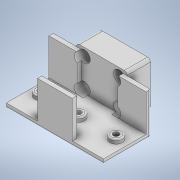
# Autodesk Inventor part: bedMount
Saved by Autodesk Inventor 2020 (Build 240168000, 168)
## iProperties
Created: 2020-01-08
Part Number: bedMount
Material: Generic
Document SubType Name: Modeling
Designer: PAB
Density: 1 g/cm^3
Appearance: Default
Author: PAB
Autodesk Inventor part; units mm, degrees
ref_plane "YZ Plane" through (0, 0, 0) normal (1, 0, 0) x (0, 1, 0)
ref_plane "XZ Plane" through (0, 0, 0) normal (0, 1, 0) x (-1, 0, 0)
ref_plane "XY Plane" through (0, 0, 0) normal (0, 0, 1) x (1, 0, 0)
sketch "Sketch1" plane through (0, 0, 0) normal (0, 1, 0) x (-1, 0, 0)
  line L0 (20.5, 16.2) -> (-20.5, 16.2)
  line L1 (-20.5, 16.2) -> (-20.5, -16.2)
  line L2 (-20.5, -16.2) -> (20.5, -16.2)
  line L3 (20.5, -16.2) -> (20.5, 16.2)
  point P0 (0, 0)
  dimension "d0" = 41
  dimension "d1" = 32.4
  constraints: 8 end point, 2 parallel, 1 horizontal, 1 perpendicular
  measures "d0" distance of L2.end L1.end
  measures "d1" distance of L1.end L0.end
extrude "Extrusion1" add sketch "Sketch1" along normal blind 3
sketch "Sketch3" plane through (0, 3, 0) normal (0, 1, 0) x (1, 0, 0)
  line L0 (-20.5, -16.2) -> (20.5, -16.2) projected
  line L1 (-20.5, 16.2) -> (-20.5, -16.2) projected
  line L2 (20.5, -16.2) -> (-20.5, -16.2)
  line L3 (-20.5, -16.2) -> (-20.5, -13.2)
  line L4 (-20.5, -13.2) -> (20.5, -13.2)
  line L5 (20.5, -13.2) -> (20.5, -16.2)
  line L6 (20.5, 16.2) -> (-20.5, 16.2) projected
  line L7 (20.5, 16.2) -> (-20.5, 16.2)
  line L8 (-20.5, 16.2) -> (-20.5, 13.2)
  line L9 (-20.5, 13.2) -> (20.5, 13.2)
  line L10 (20.5, 13.2) -> (20.5, 16.2)
  point P0 (0, 0)
  dimension "d8" = 3
  dimension "d9" = 3
  constraints: 16 end point, 4 parallel, 2 horizontal, 2 perpendicular, 2 point on line
  measures "d8" distance of L2.end L3.end
  measures "d9" distance of L8.end L7.end
extrude "Extrusion3" add sketch "Sketch3" along normal blind 25.4
sketch "Sketch4" plane through (20.5, 0, -16.2) normal (0, 0, -1) x (-1, 0, 0)
  line L0 (41, 3) -> (0, 3) projected
  line L1 (0, 28.4) -> (41, 28.4) projected
  line L2 (0, 3) -> (21.5, 3)
  line L3 (21.5, 3) -> (21.5, 28.4)
  line L4 (21.5, 28.4) -> (0, 28.4)
  line L5 (0, 28.4) -> (0, 3)
  point P0 (20.5, 0)
  dimension "d12" = 21.5
  constraints: 8 end point, 2 parallel, 1 horizontal, 1 perpendicular, 1 point on line
  measures "d12" distance of L4.end L3.end
extrude "Extrusion4" cut sketch "Sketch4" against normal blind 3
sketch "Sketch5" plane through (-20.5, 0, 16.2) normal (0, 0, 1) x (1, 0, 0)
  line L0 (41, 28.4) -> (0, 28.4) projected
  line L1 (19.5, 3) -> (41, 3) projected
  line L2 (0, 28.4) -> (21.5, 28.4)
  line L3 (21.5, 28.4) -> (21.5, 3)
  line L4 (21.5, 3) -> (0, 3)
  line L5 (0, 3) -> (0, 28.4)
  point P0 (20.5, 0)
  dimension "d15" = 21.5
  constraints: 8 end point, 2 parallel, 1 horizontal, 1 perpendicular, 1 point on line
  measures "d15" distance of L3.end L4.end
extrude "Extrusion5" cut sketch "Sketch5" against normal blind 3
sketch "Sketch6" plane through (0, 3, 0) normal (0, 1, 0) x (1, 0, 0)
  circle A0 centre (13, 0) radius 4.25
  circle A1 centre (-13, 0) radius 4.25
  line L0 (-20.5, 13.2) -> (-20.5, -16.2) projected
  line L1 (20.5, -13.2) -> (20.5, 16.2) projected
  point P0 (0, 0)
  dimension "d20" = 8.5
  dimension "d21" = 8.5
  dimension "d32" = 26
  dimension "d33" = 7.5
  dimension "d34" = 7.5
  constraints: 2 centre point
  measures "d20" diameter of A0
  measures "d21" diameter of A1
  measures "d32" distance of A0.centre A1.centre
  measures "d33" distance from line of L0 A1.centre
  measures "d34" distance from line of L1 A0.centre
extrude "Extrusion6" add sketch "Sketch6" along normal blind 3
sketch "Sketch9" plane through (20.5, 0, 16.2) normal (1, 0, 0) x (0, 0, -1)
  line L0 (32.4, 0) -> (32.4, 3) projected
  line L1 (32.4, 3) -> (0, 3)
  line L2 (0, 3) -> (0, 0)
  line L3 (0, 0) -> (32.4, 0)
  line L4 (32.4, 0) -> (32.4, 3)
  point P0 (16.2, 0)
  constraints: 8 end point, 2 parallel, 1 horizontal, 1 perpendicular
extrude "Extrusion9" add sketch "Sketch9" along normal blind 26
sketch "Sketch10" plane through (0, 3, 0) normal (0, 1, 0) x (1, 0, 0)
  circle A0 centre (39, 0) radius 4.25
  point P0 (0, 0)
  dimension "d37" = 8.5
  constraints: 1 centre point
  measures "d37" diameter of A0
extrude "Extrusion10" add sketch "Sketch10" along normal blind 3
sketch "Sketch11" plane through (0, 3, 0) normal (0, 1, 0) x (1, 0, 0)
  line L0 (46.5, 16.2) -> (46.5, -16.2) projected
  line L1 (46.5, 16.2) -> (27, 16.2)
  line L2 (27, 16.2) -> (27, 13.2)
  line L3 (27, 13.2) -> (46.5, 13.2)
  line L4 (46.5, 13.2) -> (46.5, 16.2)
  point P0 (0, 0)
  dimension "d40" = 19.5
  dimension "d41" = 3
  constraints: 8 end point, 2 parallel, 1 horizontal, 1 perpendicular
  measures "d40" distance of L3.end L2.end
  measures "d41" distance of L2.end L1.end
extrude "Extrusion11" add sketch "Sketch11" along normal blind 25.4
sketch "Sketch14" plane through (20.5, 3, 13.2) normal (1, 0, 0) x (0, 0, -1)
  line L0 (0, 0) -> (0, 25.4) projected
  line L1 (-3, 0) -> (-3, 25.4) projected
  line L2 (0, 25.4) -> (-3, 25.4)
  line L3 (-3, 25.4) -> (-3, 0)
  line L4 (-3, 0) -> (0, 0)
  line L5 (0, 0) -> (0, 25.4)
  point P0 (13.2, -3)
  constraints: 8 end point, 2 parallel, 1 horizontal, 1 perpendicular
extrude "Extrusion14" add sketch "Sketch14" along normal blind 4.5
fillet "Fillet1" radius 1 3 edges at (-17.25, 6, 0) (8.75, 6, 0) (34.75, 6, 0)
fillet "Fillet2" radius 1 6 edges at (-20.5, 14.2, -16.2) (-20.5, 0, 0) (13, 0, 16.2) (46.5, 0, 0) (46.5, 14.2, -16.2) (13, 0, -16.2)
sketch "Sketch15" plane through (0, 0, 0) normal (0, -1, 0) x (1, 0, 0)
  circle A0 centre (39, 0) radius 4.25 projected
  circle A1 centre (39, 0) radius 2
  circle A2 centre (13, 0) radius 3.25 projected
  circle A3 centre (13, 0) radius 2
  circle A4 centre (-13, 0) radius 3.25 projected
  circle A5 centre (-13, 0) radius 2
  point P0 (0, 0)
  dimension "d54" = 4
  dimension "d55" = 4
  dimension "d56" = 4
  constraints: 3 centre point, 3 coincident
  measures "d54" diameter of A1
  measures "d55" diameter of A3
  measures "d56" diameter of A5
extrude "Extrusion15" cut sketch "Sketch15" against normal blind 10 contours A1 | A3 | A5
sketch "Sketch16" plane through (0, 0, 0) normal (0, -1, 0) x (1, 0, 0)
  circle A0 centre (39, 0) radius 2 projected
  circle A1 centre (39, 0) radius 3
  circle A2 centre (13, 0) radius 2 projected
  circle A3 centre (13, 0) radius 3
  circle A4 centre (-13, 0) radius 2 projected
  circle A5 centre (-13, 0) radius 3
  point P0 (0, 0)
  dimension "d59" = 6
  dimension "d60" = 6
  dimension "d61" = 6
  constraints: 3 centre point, 3 coincident
  measures "d59" diameter of A1
  measures "d60" diameter of A3
  measures "d61" diameter of A5
extrude "Extrusion16" cut sketch "Sketch16" against normal blind 3 contours A0 | A1 | A2 | A3 | A4 | A5
sketch "Sketch17" plane through (-1, 3, -16.2) normal (0, 0, -1) x (-1, 0, 0)
  line L0 (3.5, 27.7) -> (-31.5, 27.7)
  line L1 (-31.5, 27.7) -> (-31.5, -2.3)
  line L2 (-31.5, -2.3) -> (3.5, -2.3)
  line L3 (3.5, -2.3) -> (3.5, 27.7)
  point P0 (-1, -3)
  dimension "d64" = 35
  dimension "d65" = 30
  constraints: 8 end point, 2 parallel, 1 horizontal, 1 perpendicular
  measures "d64" distance of L2.end L1.end
  measures "d65" distance of L1.end L0.end
extrude "Extrusion17" add sketch "Sketch17" along normal blind 16
sketch "Sketch18" plane through (-1, 3, -32.2) normal (0, 0, -1) x (-1, 0, 0)
  line L0 (-31.5, -2) -> (-31.5, -2.3) projected
  line L1 (0, 0) -> (19.5, 0) projected
  line L2 (-31.5, -2.3) -> (3.5, -2.3)
  line L3 (3.5, -2.3) -> (3.5, 0)
  line L4 (3.5, 0) -> (-31.5, 0)
  line L5 (-31.5, 0) -> (-31.5, -2.3)
  point P0 (-1, -3)
  dimension "d68" = 35
  constraints: 8 end point, 2 parallel, 1 horizontal, 1 perpendicular, 1 point on line
  measures "d68" distance of L4.end L3.end
extrude "Extrusion19" add sketch "Sketch18" against normal blind 19
sketch "Sketch19" plane through (-20.5, 3, -13.2) normal (0, 0, 1) x (1, 0, 0)
  circle A0 centre (45.5, 22.35) radius 4
  circle A1 centre (21.5, 22.35) radius 4
  line L0 (45.5, 25.4) -> (45.5, 0) projected
  circle A2 centre (45.5, 3.35) radius 4
  line L1 (21.5, 0) -> (21.5, 25.4) projected
  circle A3 centre (21.5, 3.35) radius 4
  point P0 (20.5, -3)
  dimension "d73" = 8
  dimension "d74" = 8
  dimension "d75" = 8
  dimension "d76" = 8
  constraints: 4 centre point, 2 point on line
  measures "d73" diameter of A0
  measures "d74" diameter of A1
  measures "d75" diameter of A2
  measures "d76" diameter of A3
extrude "Extrusion20" cut sketch "Sketch19" against normal blind 16
sketch "Sketch20" plane through (-20.5, 3, -29.2) normal (0, 0, 1) x (1, 0, 0)
  line L0 (21.5, 0) -> (21.5, 25.4) projected
  circle A0 centre (21.5, 22.225) radius 5
  arc A1 (47.5, 18.8859) -> (48.088, 25.4) centre (45.5, 22.35) ccw projected
  circle A2 centre (45.5, 22.35) radius 5
  line L1 (45.5, 25.4) -> (45.5, 0) projected
  circle A3 centre (45.5, 3.175) radius 5
  arc A4 (16, 9.1595) -> (15.5521, -2) centre (21.5, 3.35) ccw projected
  circle A5 centre (21.5, 3.35) radius 5
  point P0 (20.5, -3)
  dimension "d79" = 10
  dimension "d80" = 10
  dimension "d81" = 10
  dimension "d82" = 10
  constraints: 4 centre point, 2 coincident, 2 point on line
  measures "d79" diameter of A0
  measures "d80" diameter of A2
  measures "d81" diameter of A3
  measures "d82" diameter of A5
extrude "Extrusion21" add sketch "Sketch20" along normal blind 6
sketch "Sketch21" plane through (-1, 3, -32.2) normal (0, 0, -1) x (-1, 0, 0)
  arc A0 (-31.5, 16.8899) -> (-20.3929, 27.7) centre (-26, 22.35) ccw projected
  circle A1 centre (-26, 22.35) radius 2.75
  circle A2 centre (-2, 22.225) radius 5 projected
  circle A3 centre (-2, 22.225) radius 2.75
  circle A4 centre (-2, 3.35) radius 5 projected
  circle A5 centre (-2, 3.35) radius 2.75
  circle A6 centre (-26, 3.175) radius 5 projected
  circle A7 centre (-26, 3.175) radius 2.75
  point P0 (-1, -3)
  dimension "d85" = 5.5
  dimension "d86" = 5.5
  dimension "d87" = 5.5
  dimension "d88" = 5.5
  constraints: 4 centre point, 4 coincident, 1 other
  measures "d85" diameter of A1
  measures "d86" diameter of A3
  measures "d87" diameter of A5
  measures "d88" diameter of A7
extrude "Extrusion22" cut sketch "Sketch21" against normal blind 40 contours A1 | A3 | A5 | A7
fillet "Fillet5" radius 2 4 edges at (-4.5, 30.7, -24.2) (30.5, 30.7, -24.2) (-4.5, 0.7, -24.177) (30.5, 0.7, -24.177)
body "Solid1"
